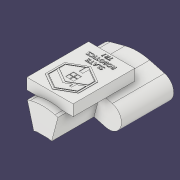
# Autodesk Inventor part: Body
Saved by Autodesk Inventor 2017 SP1 (Build 210196100, 196)
## iProperties
Created: 2018-03-03
Part Number: Body
Material: Generic
Document SubType Name: Modeling
Designer: Zach
Density: 1 g/cm^3
Appearance: CR White
Author: Zach
Autodesk Inventor part; units mm, degrees
ref_plane "YZ Plane" through (0, 0, 0) normal (1, 0, 0) x (0, 1, 0)
ref_plane "XZ Plane" through (0, 0, 0) normal (0, 1, 0) x (-1, 0, 0)
sketch "Sketch1" plane through (0, 0, 0) normal (0, 0, 1) x (1, 0, 0)
  line L0 (106.5, -56.5) -> (106.5, 56.5)
  line L1 (38.589, -78.0481) -> (135.1815, -103.93)
  circle A0 centre (155.8871, -26.656) radius 5.25
  line L2 (80, 76.5) -> (176.5926, 50.6181)
  circle A1 centre (155.8871, -26.656) radius 80 construction
  arc A2 (135.1815, -103.93) -> (176.5926, 50.6181) centre (155.8871, -26.656) ccw
  circle A3 centre (-155.8871, -26.656) radius 80 construction
  line L3 (-176.5926, 50.6181) -> (-80, 76.5)
  circle A4 centre (-155.8871, -26.656) radius 5.25
  arc A5 (-176.5926, 50.6181) -> (-135.1815, -103.93) centre (-155.8871, -26.656) ccw
  line L4 (-106.5, 56.5) -> (-106.5, -56.5)
  line L5 (80, 76.5) -> (38.589, -78.0481) construction
  circle A6 centre (0, 71.664) radius 5.25
  line L6 (-38.589, -78.0481) -> (38.589, -78.0481)
  line L7 (-80, 76.5) -> (-38.589, -78.0481) construction
  line L8 (-135.1815, -103.93) -> (-38.589, -78.0481)
  line L9 (-106.5, -56.5) -> (106.5, -56.5)
  line L10 (106.5, 56.5) -> (-106.5, 56.5)
  line L11 (-80, 76.5) -> (80, 76.5) construction
  arc A7 (80, 76.5) -> (-80, 76.5) centre (0, -228.172) ccw
  line L12 (310, 185.5) -> (-310, 185.5) construction
  line L13 (0, 185.5) -> (0, 0) construction
  line L14 (0, 0) -> (310, 0) construction
  line L15 (310, 75.5) -> (310, -324.5) construction
  line L16 (0, -78.0481) -> (0, -56.5)
  point P0 (0, 0)
  point P1 (0, 76.5)
  point P2 (-106.5, 0)
  dimension "d0" = 160
  dimension "d1" = 100
  dimension "d2" = 100
  dimension "d3" = 160
  dimension "d4" = 160
  dimension "d5" = 160
  dimension "d6" = 75
  dimension "d7" = 75
  dimension "d8" = 160
  dimension "d9" = 100
  dimension "d10" = 100
  dimension "d11" = 10.5
  dimension "d12" = 10.5
  dimension "d13" = 113
  dimension "d14" = 213
  dimension "d15" = 20
  dimension "d16" = 315
  dimension "d17" = 10.5
  dimension "d18" = 15.164
  dimension "d19" = 185.5
  constraints: 34 end point, 10 point on circle, 8 centre point, 8 tangent, 5 coincident, 5 midpoint, 3 perpendicular, 2 parallel, 2 point on line, 2 vertical alignment, 1 horizontal alignment, 1 vertical
  measures "d0" diameter of A3
  measures "d1" distance of L11.start L3.start
  measures "d2" distance of L6.start L8.start
  measures "d3" distance of L11.start L6.start
  measures "d4" distance of L11.start L11.end
  measures "d5" distance of L11.end L6.end
  measures "d6" angle of L11 L7
  measures "d7" angle of L11 L5
  measures "d8" diameter of A1
  measures "d9" distance of L6.end L1.end
  measures "d10" distance of L11.end L2.end
  measures "d11" diameter of A4
  measures "d12" diameter of A0
  measures "d13" distance of L10.start L9.end
  measures "d14" distance of L9.end L9.start
  measures "d15" distance between parallel lines of L11 L10
  measures "d16" radius of A7
  measures "d17" diameter of A6
  measures "d18" distance from line of L10 A6.centre
  measures "d19" distance of L13.start L13.end
extrude "Extrusion1" add sketch "Sketch1" along normal blind 70 and the other way blind 269 contours L9 L4 L10 L0 | L6 L8 A5 L3 A7 L2 A2 L1 | A0 | A4 | A6
sketch "Sketch2" plane through (0, 0, 70) normal (0, 0, 1) x (1, 0, 0)
  line L0 (-38.589, -78.0481) -> (38.589, -78.0481) projected
  line L1 (-176.5926, 50.6181) -> (-80, 76.5) projected
  line L2 (-38.589, -78.0481) -> (-80, 76.5)
  line L3 (176.5926, 50.6181) -> (80, 76.5) projected
  line L4 (38.589, -78.0481) -> (80, 76.5)
  arc A0 (80, 76.5) -> (-80, 76.5) centre (0, -228.172) ccw projected
  point P0 (0, 0)
  constraints: 4 end point, 2 perpendicular
extrude "Extrusion2" add sketch "Sketch2" along normal blind 275
ref_plane "Work Plane1" through (-38.589, 76.9519, -269) normal (0, -1, 0) x (1, 0, 0)
sketch "Sketch3" plane through (-38.589, 76.9519, -269) normal (0, -1, 0) x (1, 0, 0)
  line L0 (188.589, 566.5) -> (-111.411, 566.5)
  line L1 (-111.411, 566.5) -> (-111.411, 166.5)
  line L2 (-111.411, 166.5) -> (188.589, 166.5)
  line L3 (188.589, 166.5) -> (188.589, 566.5)
  line L4 (118.589, 614) -> (-41.411, 614) projected
  point P0 (38.589, 269)
  point P1 (38.589, 566.5)
  point P2 (38.589, 614)
  dimension "d25" = 300
  dimension "d26" = 400
  dimension "d27" = 47.5
  constraints: 8 end point, 2 midpoint, 2 parallel, 1 horizontal, 1 perpendicular, 1 vertical alignment
  measures "d25" distance of L2.end L1.end
  measures "d26" distance of L1.end L0.end
  measures "d27" distance between parallel lines of L4 L0
extrude "Extrusion3" add sketch "Sketch3" against normal blind 72
sketch "Sketch4" plane through (-38.589, 148.9519, -269) normal (0, 1, 0) x (1, 0, 0)
  line L0 (188.589, -301.5) -> (-111.411, -301.5) construction
  line L1 (-111.411, -301.5) -> (-111.411, -166.5) construction
  line L2 (-111.411, -166.5) -> (188.589, -166.5) construction
  line L3 (188.589, -166.5) -> (188.589, -301.5) construction
  line L4 (163.589, -551.5) -> (-86.411, -551.5) construction
  line L5 (-86.411, -551.5) -> (-86.411, -301.5) construction
  line L6 (-86.411, -301.5) -> (163.589, -301.5) construction
  line L7 (163.589, -301.5) -> (163.589, -551.5) construction
  line L8 (-111.411, -566.5) -> (188.589, -566.5)
  line L9 (-111.411, -166.5) -> (-111.411, -566.5)
  line L10 (38.589, -551.5) -> (-69.6642, -489)
  line L11 (-69.6642, -489) -> (-69.6642, -364)
  line L12 (-69.6642, -364) -> (38.589, -301.5)
  line L13 (38.589, -301.5) -> (146.8421, -364)
  line L14 (146.8421, -364) -> (146.8421, -489)
  line L15 (146.8421, -489) -> (38.589, -551.5)
  line L16 (38.589, -539.7221) -> (-59.4642, -483.111)
  line L17 (-59.4642, -483.111) -> (-59.4642, -369.889)
  line L18 (-59.4642, -369.889) -> (38.589, -313.2779)
  line L19 (38.589, -313.2779) -> (136.6421, -369.889)
  line L20 (136.6421, -369.889) -> (136.6421, -483.111)
  line L21 (136.6421, -483.111) -> (38.589, -539.7221)
  line L22 (38.589, -534.8146) -> (-55.2142, -480.6573) construction
  line L23 (-55.2142, -480.6573) -> (-55.2142, -372.3427) construction
  line L24 (-55.2142, -372.3427) -> (38.589, -318.1854) construction
  line L25 (38.589, -318.1854) -> (132.3921, -372.3427) construction
  line L26 (132.3921, -372.3427) -> (132.3921, -480.6573) construction
  line L27 (132.3921, -480.6573) -> (38.589, -534.8146) construction
  line L28 (132.3921, -428.1573) -> (92.3921, -451.2513)
  line L29 (92.3921, -451.2513) -> (92.3921, -479.7513)
  line L30 (92.3921, -479.7513) -> (78.3921, -479.7513)
  line L31 (78.3921, -479.7513) -> (78.3921, -459.3342)
  line L32 (78.3921, -459.3342) -> (38.589, -482.3146)
  line L33 (38.589, -482.3146) -> (-55.2142, -428.1573)
  line L34 (-55.2142, -428.1573) -> (-55.2142, -480.6573)
  line L35 (-55.2142, -480.6573) -> (38.589, -534.8146)
  line L36 (38.589, -534.8146) -> (132.3921, -480.6573)
  line L37 (132.3921, -428.1573) -> (132.3921, -480.6573)
  line L38 (132.3921, -372.3427) -> (50.589, -325.1136)
  line L39 (50.589, -325.1136) -> (50.589, -365.1854)
  line L40 (50.589, -365.1854) -> (26.589, -365.1854)
  line L41 (26.589, -365.1854) -> (26.589, -325.1136)
  line L42 (26.589, -325.1136) -> (-55.2142, -372.3427)
  line L43 (-55.2142, -372.3427) -> (-55.2142, -413.1573)
  line L44 (-55.2142, -413.1573) -> (38.589, -467.3146)
  line L45 (38.589, -467.3146) -> (132.3921, -413.1573)
  line L46 (132.3921, -413.1573) -> (132.3921, -372.3427)
  line L47 (64.839, -439.1854) -> (12.339, -439.1854) construction
  line L48 (12.339, -439.1854) -> (12.339, -388.1854) construction
  line L49 (12.339, -388.1854) -> (64.839, -388.1854) construction
  line L50 (64.839, -388.1854) -> (64.839, -439.1854) construction
  line L51 (64.839, -388.1854) -> (40.839, -388.1854)
  line L52 (40.839, -388.1854) -> (40.839, -412.1854)
  line L53 (40.839, -412.1854) -> (64.839, -412.1854)
  line L54 (64.839, -412.1854) -> (64.839, -388.1854)
  line L55 (64.839, -439.1854) -> (40.839, -439.1854)
  line L56 (40.839, -439.1854) -> (40.839, -415.1854)
  line L57 (40.839, -415.1854) -> (64.839, -415.1854)
  line L58 (64.839, -415.1854) -> (64.839, -439.1854)
  line L59 (12.339, -439.1854) -> (36.339, -439.1854)
  line L60 (36.339, -439.1854) -> (36.339, -415.1854)
  line L61 (36.339, -415.1854) -> (12.339, -415.1854)
  line L62 (12.339, -415.1854) -> (12.339, -439.1854)
  line L63 (12.339, -388.1854) -> (36.339, -388.1854)
  line L64 (36.339, -388.1854) -> (36.339, -412.1854)
  line L65 (36.339, -412.1854) -> (12.339, -412.1854)
  line L66 (12.339, -412.1854) -> (12.339, -388.1854)
  line L67 (38.589, -566.5) -> (38.589, -551.5)
  line L68 (38.589, -551.5) -> (38.589, -301.5) construction
  line L69 (188.589, -166.5) -> (-111.411, -166.5) projected
  line L70 (91.8407, -261.3958) -> (91.8407, -265.6804)
  spline S0 degree 2 poles (91.8407, -265.6804) (88.9141, -264.4563) (86.0258, -263.9781) (84.8208, -263.9781) knots 0 0 0 1 2 2 2
  spline S1 degree 2 poles (84.8208, -263.9781) (82.6402, -263.9781) (80.4788, -265.9291) (80.4788, -267.3063) knots 0 0 0 1 2 2 2
  spline S2 degree 2 poles (80.4788, -267.3063) (80.4788, -268.3583) (81.0717, -269.2) knots 0 0 0 1 1 1
  spline S3 degree 2 poles (81.0717, -269.2) (81.6838, -270.0224) (84.0365, -271.3423) knots 0 0 0 1 1 1
  line L71 (84.0365, -271.3423) -> (85.7198, -272.2795)
  spline S4 degree 2 poles (85.7198, -272.2795) (89.3349, -274.2879) (90.5974, -275.9903) knots 0 0 0 1 1 1
  spline S5 degree 2 poles (90.5974, -275.9903) (91.8981, -277.6927) (91.8981, -279.9306) knots 0 0 0 1 1 1
  spline S6 degree 2 poles (91.8981, -279.9306) (91.8981, -282.7615) (87.5752, -286.7784) (83.5392, -286.7784) knots 0 0 0 1 2 2 2
  spline S7 degree 2 poles (83.5392, -286.7784) (80.517, -286.7784) (76.7297, -285.9176) knots 0 0 0 1 1 1
  line L72 (76.7297, -285.9176) -> (76.7297, -281.9199)
  spline S8 degree 2 poles (76.7297, -281.9199) (80.6127, -283.3545) (82.8889, -283.3545) knots 0 0 0 1 1 1
  spline S9 degree 2 poles (82.8889, -283.3545) (84.7825, -283.3545) (86.7527, -281.7095) (86.7527, -280.5618) knots 0 0 0 1 2 2 2
  spline S10 degree 2 poles (86.7527, -280.5618) (86.7527, -279.682) (86.1406, -278.936) knots 0 0 0 1 1 1
  spline S11 degree 2 poles (86.1406, -278.936) (85.5668, -278.1709) (83.214, -276.8511) knots 0 0 0 1 1 1
  line L73 (83.214, -276.8511) -> (81.416, -275.8564)
  spline S12 degree 2 poles (81.416, -275.8564) (77.2653, -273.542) (76.1368, -271.8396) knots 0 0 0 1 1 1
  spline S13 degree 2 poles (76.1368, -271.8396) (75.0082, -270.1181) (75.0082, -267.9758) knots 0 0 0 1 1 1
  spline S14 degree 2 poles (75.0082, -267.9758) (75.0082, -264.8962) (79.6945, -260.5542) (84.8017, -260.5542) knots 0 0 0 1 2 2 2
  spline S15 degree 2 poles (84.8017, -260.5542) (87.8238, -260.5542) (91.8407, -261.3958) knots 0 0 0 1 1 1
  line L74 (70.6854, -261.1663) -> (70.6854, -286.1663)
  line L75 (70.6854, -286.1663) -> (65.4826, -286.1663)
  line L76 (65.4826, -286.1663) -> (65.4826, -264.7049)
  line L77 (65.4826, -264.7049) -> (54.3311, -264.7049)
  line L78 (54.3311, -264.7049) -> (54.3311, -261.1663)
  line L79 (54.3311, -261.1663) -> (70.6854, -261.1663)
  line L80 (53.3173, -261.1663) -> (43.6196, -286.1663)
  line L81 (43.6196, -286.1663) -> (38.3977, -286.1663)
  line L82 (38.3977, -286.1663) -> (28.6616, -261.1663)
  line L83 (28.6616, -261.1663) -> (33.9983, -261.1663)
  line L84 (33.9983, -261.1663) -> (36.5997, -267.8419)
  line L85 (36.5997, -267.8419) -> (46.9287, -267.8419)
  line L86 (46.9287, -267.8419) -> (49.53, -261.1663)
  line L87 (49.53, -261.1663) -> (53.3173, -261.1663)
  line L88 (45.6471, -271.1701) -> (37.9004, -271.1701)
  line L89 (37.9004, -271.1701) -> (41.7642, -281.1357)
  line L90 (41.7642, -281.1357) -> (45.6471, -271.1701)
  line L91 (18.9065, -261.1663) -> (18.9065, -282.7233)
  line L92 (18.9065, -282.7233) -> (27.8583, -282.7233)
  line L93 (27.8583, -282.7233) -> (27.8583, -286.1663)
  line L94 (27.8583, -286.1663) -> (4.7519, -286.1663)
  line L95 (4.7519, -286.1663) -> (4.7519, -282.7233)
  line L96 (4.7519, -282.7233) -> (13.7037, -282.7233)
  line L97 (13.7037, -282.7233) -> (13.7037, -261.1663)
  line L98 (13.7037, -261.1663) -> (18.9065, -261.1663)
  line L99 (1.2707, -261.1663) -> (1.2707, -286.1663)
  line L100 (1.2707, -286.1663) -> (-14.7393, -286.1663)
  line L101 (-14.7393, -286.1663) -> (-14.7393, -282.7233)
  line L102 (-14.7393, -282.7233) -> (-3.9321, -282.7233)
  line L103 (-3.9321, -282.7233) -> (-3.9321, -275.7608)
  line L104 (-3.9321, -275.7608) -> (-12.8648, -275.7608)
  line L105 (-12.8648, -275.7608) -> (-12.8648, -272.3178)
  line L106 (-12.8648, -272.3178) -> (-3.9321, -272.3178)
  line L107 (-3.9321, -272.3178) -> (-3.9321, -264.7049)
  line L108 (-3.9321, -264.7049) -> (-15.5426, -264.7049)
  line L109 (-15.5426, -264.7049) -> (-15.5426, -261.1663)
  line L110 (-15.5426, -261.1663) -> (1.2707, -261.1663)
  line L111 (126.6054, -221.2098) -> (126.6054, -246.2098)
  line L112 (126.6054, -246.2098) -> (117.2519, -246.2098)
  spline S16 degree 2 poles (117.2519, -246.2098) (114.3828, -246.2098) (111.3797, -244.7752) (109.6391, -241.8486) (109.6391, -240.0124) knots 0 0 0 1 2 3 3 3
  spline S17 degree 2 poles (109.6391, -240.0124) (109.6391, -237.8127) (112.1639, -233.9106) (114.4784, -232.8777) knots 0 0 0 1 2 2 2
  line L113 (114.4784, -232.8777) -> (106.3108, -221.2098)
  line L114 (106.3108, -221.2098) -> (112.6421, -221.2098)
  line L115 (112.6421, -221.2098) -> (118.8586, -231.424)
  line L116 (118.8586, -231.424) -> (121.7087, -231.424)
  line L117 (121.7087, -231.424) -> (121.7087, -221.2098)
  line L118 (121.7087, -221.2098) -> (126.6054, -221.2098)
  line L119 (121.7087, -234.8479) -> (120.5228, -234.8479)
  spline S18 degree 2 poles (120.5228, -234.8479) (117.3093, -234.8479) (114.8418, -237.6597) (114.8418, -239.4385) knots 0 0 0 1 2 2 2
  spline S19 degree 2 poles (114.8418, -239.4385) (114.8418, -240.9688) (116.8311, -242.7859) (119.8915, -242.7859) knots 0 0 0 1 2 2 2
  line L120 (119.8915, -242.7859) -> (121.7087, -242.7859)
  line L121 (121.7087, -242.7859) -> (121.7087, -234.8479)
  spline S20 degree 2 poles (91.6207, -220.5977) (95.5228, -220.5977) (101.2994, -223.8303) (104.3024, -229.8747) (104.3024, -233.7193) knots 0 0 0 1 2 3 3 3
  spline S21 degree 2 poles (104.3024, -233.7193) (104.3024, -237.5258) (101.2994, -243.6084) (95.4845, -246.8219) (91.6207, -246.8219) knots 0 0 0 1 2 3 3 3
  spline S22 degree 2 poles (91.6207, -246.8219) (87.776, -246.8219) (81.9612, -243.6084) (78.9581, -237.5258) (78.9581, -233.7193) knots 0 0 0 1 2 3 3 3
  spline S23 degree 2 poles (78.9581, -233.7193) (78.9581, -229.8747) (81.9612, -223.8303) (87.7186, -220.5977) (91.6207, -220.5977) knots 0 0 0 1 2 3 3 3
  spline S24 degree 2 poles (91.6207, -224.0216) (88.0056, -224.0216) (84.486, -229.9129) (84.486, -233.7193) knots 0 0 0 1 2 2 2
  spline S25 degree 2 poles (84.486, -233.7193) (84.486, -237.5449) (88.0247, -243.398) (91.6207, -243.398) knots 0 0 0 1 2 2 2
  spline S26 degree 2 poles (91.6207, -243.398) (95.2358, -243.398) (98.7745, -237.5449) (98.7745, -233.7193) knots 0 0 0 1 2 2 2
  spline S27 degree 2 poles (98.7745, -233.7193) (98.7745, -229.9129) (95.255, -224.0216) (91.6207, -224.0216) knots 0 0 0 1 2 2 2
  line L122 (74.2909, -221.2098) -> (74.2909, -246.2098)
  line L123 (74.2909, -246.2098) -> (65.8556, -246.2098)
  spline S28 degree 2 poles (65.8556, -246.2098) (62.7951, -246.2098) (59.8686, -244.8326) (58.2045, -242.1547) (58.2045, -240.6436) knots 0 0 0 1 2 3 3 3
  spline S29 degree 2 poles (58.2045, -240.6436) (58.2045, -238.7691) (60.8059, -235.3261) (64.1723, -234.274) knots 0 0 0 1 2 2 2
  spline S30 degree 2 poles (64.1723, -234.274) (61.4945, -233.6046) (58.6635, -231.6535) (57.1907, -228.9374) (57.1907, -227.388) knots 0 0 0 1 2 3 3 3
  spline S31 degree 2 poles (57.1907, -227.388) (57.1907, -225.7048) (58.9122, -222.7783) (61.9344, -221.2098) (65.0713, -221.2098) knots 0 0 0 1 2 3 3 3
  line L124 (65.0713, -221.2098) -> (74.2909, -221.2098)
  line L125 (69.2986, -224.7484) -> (68.3039, -224.7484)
  spline S32 degree 2 poles (68.3039, -224.7484) (65.5878, -224.7484) (63.6176, -225.4561) (62.623, -227.0437) (62.623, -228.0193) knots 0 0 0 1 2 3 3 3
  spline S33 degree 2 poles (62.623, -228.0193) (62.623, -229.8747) (65.8938, -232.4569) (68.3996, -232.4569) knots 0 0 0 1 2 2 2
  line L126 (68.3996, -232.4569) -> (69.2986, -232.4569)
  line L127 (69.2986, -232.4569) -> (69.2986, -224.7484)
  line L128 (69.2986, -235.8043) -> (68.1892, -235.8043)
  spline S34 degree 2 poles (68.1892, -235.8043) (65.8173, -235.8043) (63.4837, -238.157) (63.4837, -239.8402) knots 0 0 0 1 2 2 2
  spline S35 degree 2 poles (63.4837, -239.8402) (63.4837, -240.7392) (64.1723, -242.0591) (65.913, -242.7859) (68.3613, -242.7859) knots 0 0 0 1 2 3 3 3
  line L129 (68.3613, -242.7859) -> (69.2986, -242.7859)
  line L130 (69.2986, -242.7859) -> (69.2986, -235.8043)
  spline S36 degree 2 poles (41.372, -220.5977) (45.2741, -220.5977) (51.0507, -223.8303) (54.0538, -229.8747) (54.0538, -233.7193) knots 0 0 0 1 2 3 3 3
  spline S37 degree 2 poles (54.0538, -233.7193) (54.0538, -237.5258) (51.0507, -243.6084) (45.2358, -246.8219) (41.372, -246.8219) knots 0 0 0 1 2 3 3 3
  spline S38 degree 2 poles (41.372, -246.8219) (37.5274, -246.8219) (31.7125, -243.6084) (28.7095, -237.5258) (28.7095, -233.7193) knots 0 0 0 1 2 3 3 3
  spline S39 degree 2 poles (28.7095, -233.7193) (28.7095, -229.8747) (31.7125, -223.8303) (37.47, -220.5977) (41.372, -220.5977) knots 0 0 0 1 2 3 3 3
  spline S40 degree 2 poles (41.372, -224.0216) (37.7569, -224.0216) (34.2374, -229.9129) (34.2374, -233.7193) knots 0 0 0 1 2 2 2
  spline S41 degree 2 poles (34.2374, -233.7193) (34.2374, -237.5449) (37.776, -243.398) (41.372, -243.398) knots 0 0 0 1 2 2 2
  spline S42 degree 2 poles (41.372, -243.398) (44.9872, -243.398) (48.5258, -237.5449) (48.5258, -233.7193) knots 0 0 0 1 2 2 2
  spline S43 degree 2 poles (48.5258, -233.7193) (48.5258, -229.9129) (45.0063, -224.0216) (41.372, -224.0216) knots 0 0 0 1 2 2 2
  line L131 (17.8257, -221.2098) -> (17.8257, -242.7668)
  line L132 (17.8257, -242.7668) -> (26.7775, -242.7668)
  line L133 (26.7775, -242.7668) -> (26.7775, -246.2098)
  line L134 (26.7775, -246.2098) -> (3.6712, -246.2098)
  line L135 (3.6712, -246.2098) -> (3.6712, -242.7668)
  line L136 (3.6712, -242.7668) -> (12.623, -242.7668)
  line L137 (12.623, -242.7668) -> (12.623, -221.2098)
  line L138 (12.623, -221.2098) -> (17.8257, -221.2098)
  line L139 (0.1899, -221.2098) -> (0.1899, -246.2098)
  line L140 (0.1899, -246.2098) -> (-5.0128, -246.2098)
  line L141 (-5.0128, -246.2098) -> (-5.0128, -221.2098)
  line L142 (-5.0128, -221.2098) -> (0.1899, -221.2098)
  spline S44 degree 2 poles (-31.39, -222.2044) (-29.745, -221.4776) (-27.3158, -220.942) (-24.2362, -220.5977) (-22.7251, -220.5977) knots 0 0 0 1 2 3 3 3
  spline S45 degree 2 poles (-22.7251, -220.5977) (-16.1643, -220.5977) (-9.7182, -227.981) (-9.7182, -233.7193) knots 0 0 0 1 2 2 2
  spline S46 degree 2 poles (-9.7182, -233.7193) (-9.7182, -239.4577) (-16.1452, -246.8219) (-23.0503, -246.8219) knots 0 0 0 1 2 2 2
  spline S47 degree 2 poles (-23.0503, -246.8219) (-27.1245, -246.8219) (-31.1605, -245.8655) knots 0 0 0 1 1 1
  line L143 (-31.1605, -245.8655) -> (-31.1605, -241.7913)
  spline S48 degree 2 poles (-31.1605, -241.7913) (-29.2094, -242.4607) (-26.742, -243.092) (-24.5423, -243.398) (-23.4329, -243.398) knots 0 0 0 1 2 3 3 3
  spline S49 degree 2 poles (-23.4329, -243.398) (-19.1291, -243.398) (-15.2462, -237.8701) (-15.2462, -233.7767) knots 0 0 0 1 2 2 2
  spline S50 degree 2 poles (-15.2462, -233.7767) (-15.2462, -229.4921) (-19.6456, -224.1937) (-24.0067, -224.1937) knots 0 0 0 1 2 2 2
  spline S51 degree 2 poles (-24.0067, -224.1937) (-27.641, -224.1937) (-31.39, -226.03) knots 0 0 0 1 1 1
  line L144 (-31.39, -226.03) -> (-31.39, -222.2044)
  line L145 (-34.5078, -221.4393) -> (-34.5078, -225.7239)
  spline S52 degree 2 poles (-34.5078, -225.7239) (-37.4344, -224.4998) (-40.3227, -224.0216) (-41.5277, -224.0216) knots 0 0 0 1 2 2 2
  spline S53 degree 2 poles (-41.5277, -224.0216) (-43.7083, -224.0216) (-45.8697, -225.9726) (-45.8697, -227.3498) knots 0 0 0 1 2 2 2
  spline S54 degree 2 poles (-45.8697, -227.3498) (-45.8697, -228.4018) (-45.2768, -229.2434) knots 0 0 0 1 1 1
  spline S55 degree 2 poles (-45.2768, -229.2434) (-44.6647, -230.0659) (-42.312, -231.3858) knots 0 0 0 1 1 1
  line L146 (-42.312, -231.3858) -> (-40.6287, -232.323)
  spline S56 degree 2 poles (-40.6287, -232.323) (-37.0136, -234.3314) (-35.7511, -236.0338) knots 0 0 0 1 1 1
  spline S57 degree 2 poles (-35.7511, -236.0338) (-34.4505, -237.7362) (-34.4505, -239.9741) knots 0 0 0 1 1 1
  spline S58 degree 2 poles (-34.4505, -239.9741) (-34.4505, -242.805) (-38.7733, -246.8219) (-42.8093, -246.8219) knots 0 0 0 1 2 2 2
  spline S59 degree 2 poles (-42.8093, -246.8219) (-45.8315, -246.8219) (-49.6188, -245.9611) knots 0 0 0 1 1 1
  line L147 (-49.6188, -245.9611) -> (-49.6188, -241.9634)
  spline S60 degree 2 poles (-49.6188, -241.9634) (-45.7358, -243.398) (-43.4596, -243.398) knots 0 0 0 1 1 1
  spline S61 degree 2 poles (-43.4596, -243.398) (-41.566, -243.398) (-39.5958, -241.753) (-39.5958, -240.6053) knots 0 0 0 1 2 2 2
  spline S62 degree 2 poles (-39.5958, -240.6053) (-39.5958, -239.7255) (-40.2079, -238.9795) knots 0 0 0 1 1 1
  spline S63 degree 2 poles (-40.2079, -238.9795) (-40.7817, -238.2144) (-43.1345, -236.8946) knots 0 0 0 1 1 1
  line L148 (-43.1345, -236.8946) -> (-44.9325, -235.8999)
  spline S64 degree 2 poles (-44.9325, -235.8999) (-49.0832, -233.5854) (-50.2117, -231.8831) knots 0 0 0 1 1 1
  spline S65 degree 2 poles (-50.2117, -231.8831) (-51.3403, -230.1616) (-51.3403, -228.0193) knots 0 0 0 1 1 1
  spline S66 degree 2 poles (-51.3403, -228.0193) (-51.3403, -224.9397) (-46.654, -220.5977) (-41.5469, -220.5977) knots 0 0 0 1 2 2 2
  spline S67 degree 2 poles (-41.5469, -220.5977) (-38.5247, -220.5977) (-34.5078, -221.4393) knots 0 0 0 1 1 1
  line L149 (62.2428, -181.2216) -> (57.7813, -203.5678)
  line L150 (57.7813, -203.5678) -> (66.6659, -203.5678)
  line L151 (66.6659, -203.5678) -> (66.1466, -206.2216)
  line L152 (66.1466, -206.2216) -> (44.8582, -206.2216)
  line L153 (44.8582, -206.2216) -> (45.3966, -203.5678)
  line L154 (45.3966, -203.5678) -> (54.262, -203.5678)
  line L155 (54.262, -203.5678) -> (58.7043, -181.2216)
  line L156 (58.7043, -181.2216) -> (62.2428, -181.2216)
  line L157 (46.4543, -181.2216) -> (41.4736, -206.2216)
  line L158 (41.4736, -206.2216) -> (33.9351, -206.2216)
  spline S68 degree 2 poles (33.9351, -206.2216) (31.9543, -206.2216) (29.2428, -205.5485) (27.4543, -203.1255) (27.4543, -201.3755) knots 0 0 0 1 2 3 3 3
  spline S69 degree 2 poles (27.4543, -201.3755) (27.4543, -198.837) (31.0697, -194.337) (34.1466, -193.1639) knots 0 0 0 1 2 2 2
  line L159 (34.1466, -193.1639) -> (28.2043, -181.2216)
  line L160 (28.2043, -181.2216) -> (32.1274, -181.2216)
  line L161 (32.1274, -181.2216) -> (37.3774, -192.2793)
  line L162 (37.3774, -192.2793) -> (40.7236, -192.2793)
  line L163 (40.7236, -192.2793) -> (42.9159, -181.2216)
  line L164 (42.9159, -181.2216) -> (46.4543, -181.2216)
  line L165 (40.2043, -194.8947) -> (38.2428, -194.8947)
  spline S70 degree 2 poles (38.2428, -194.8947) (36.1466, -194.8947) (33.0505, -196.4716) (31.2236, -199.4716) (31.2236, -200.9716) knots 0 0 0 1 2 3 3 3
  spline S71 degree 2 poles (31.2236, -200.9716) (31.2236, -202.2601) (33.1851, -203.5678) (36.2236, -203.5678) knots 0 0 0 1 2 2 2
  line L166 (36.2236, -203.5678) -> (38.4736, -203.5678)
  line L167 (38.4736, -203.5678) -> (40.2043, -194.8947)
  line L168 (18.762, -181.2216) -> (14.2813, -203.6832)
  line L169 (14.2813, -203.6832) -> (18.1851, -203.6832)
  line L170 (18.1851, -203.6832) -> (17.762, -205.7601)
  line L171 (17.762, -205.7601) -> (10.3774, -206.4332)
  line L172 (10.3774, -206.4332) -> (15.4351, -181.2216)
  line L173 (15.4351, -181.2216) -> (18.762, -181.2216)
  point P0 (38.589, -269)
  point P1 (38.589, -426.5)
  point P2 (38.589, -365.1854)
  point P3 (38.589, -439.1854)
  point P4 (38.589, -388.1854)
  point P5 (38.589, -166.5)
  dimension "d30" = 15
  dimension "d31" = 250
  dimension "d32" = 10.2
  dimension "d33" = 4.25
  dimension "d34" = 52.5
  dimension "d35" = 40
  dimension "d36" = 14
  dimension "d37" = 28.5
  dimension "d38" = 15
  dimension "d39" = 24
  dimension "d40" = 47
  dimension "d41" = 23
  dimension "d42" = 51
  dimension "d43" = 52.5
  dimension "d44" = 24
  dimension "d45" = 24
  dimension "d46" = 24
  dimension "d47" = 24
  dimension "d48" = 24
  dimension "d49" = 24
  dimension "d50" = 24
  dimension "d51" = 24
  dimension "d54" = 300
  dimension "d56" = 400
  constraints: 122 end point, 16 parallel, 16 perpendicular, 12 point on line, 9 midpoint, 4 collinear, 1 coincident, 1 horizontal, 26 other
  measures "d30" distance between parallel lines of L8 L4
  measures "d31" distance of L7.end L5.start
  measures "d32" distance between parallel lines of L15 L21
  measures "d33" distance between parallel lines of L21 L27
  measures "d34" distance of L28.start L37.end
  measures "d35" distance between parallel lines of L26 L29
  measures "d36" distance of L30.start L30.end
  measures "d37" distance of L29.start L30.start
  measures "d38" distance of L33.start L44.end
  measures "d39" distance between parallel lines of L41 L39
  measures "d40" distance from line of L24.end L40
  measures "d41" distance between parallel lines of L40 L49
  measures "d42" distance of L51.start L55.start
  measures "d43" distance of L55.start L62.end
  measures "d44" distance of L53.end L53.start
  measures "d45" distance of L53.start L51.end
  measures "d46" distance of L56.end L57.end
  measures "d47" distance of L55.end L56.end
  measures "d48" distance of L61.end L61.start
  measures "d49" distance of L61.start L60.start
  measures "d50" distance of L64.end L66.start
  measures "d51" distance of L64.start L64.end
  measures "d54" distance of L9.end L8.end
  measures "d56" distance of L9.start L9.end
extrude "Extrusion4" add sketch "Sketch4" along normal blind 2
sketch "Sketch5" plane through (0, 0, 70) normal (0, 0, 1) x (1, 0, 0)
  line L0 (-80, 76.5) -> (-38.589, -78.0481) projected
  line L1 (38.589, -78.0481) -> (80, 76.5) projected
  line L2 (-80, 76.5) -> (-99.3185, 71.3236)
  line L3 (-176.5926, 50.6181) -> (-80, 76.5) projected
  line L4 (-99.3185, 71.3236) -> (-57.9075, -83.2245)
  line L5 (-38.589, -78.0481) -> (-135.1815, -103.93) projected
  line L6 (38.589, -78.0481) -> (-38.589, -78.0481) projected
  line L7 (-38.589, -78.0481) -> (-57.9075, -83.2245)
  line L8 (80, 76.5) -> (38.589, -78.0481)
  line L9 (57.9075, -83.2245) -> (99.3185, 71.3236)
  line L10 (99.3185, 71.3236) -> (80, 76.5)
  line L11 (135.1815, -103.93) -> (38.589, -78.0481) projected
  line L12 (57.9075, -83.2245) -> (38.589, -78.0481)
  point P0 (0, 0)
  dimension "d98" = 20
  dimension "d99" = 20
  constraints: 14 end point, 2 collinear, 2 perpendicular, 2 point on line, 1 parallel
  measures "d98" distance of L0.start L2.end
  measures "d99" distance of L9.start L1.start
extrude "Extrusion5" add sketch "Sketch5" along normal blind 275
body "Solid1"
